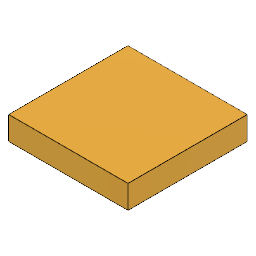
Post it Plotter v1 (Autodesk Fusion 360 archive; units mm, degrees)
design "Post It"
Autodesk Fusion 360 part; units mm, degrees
sketch "Skizze1" plane through (0, 0, 0) normal (0, 1, 0) x (1, 0, 0)
  line L0 (38.1, 38.1) -> (-38.1, 38.1)
  line L1 (-38.1, 38.1) -> (-38.1, -38.1)
  line L2 (-38.1, -38.1) -> (38.1, -38.1)
  line L3 (38.1, -38.1) -> (38.1, 38.1)
  line L4 (38.1, 38.1) -> (-38.1, -38.1) construction
  line L5 (-38.1, 38.1) -> (38.1, -38.1) construction
  dimension "d1" = 76.2
  dimension "d2" = 76.2
  constraint perpendicular L0 L1
  constraint parallel L0 L2
  constraint parallel L1 L3
  constraint horizontal L0
  constraint coincident L4 origin
  constraint coincident L5 origin
  measures "d1" distance of L1.end L2.end
  measures "d2" distance of L0.end L1.end
extrude "Extrusion1" add sketch "Skizze1" along normal blind 15 makes body 1
copy_body "Körper->Berechn1" bodies 1 removing the originals makes body 2 in component "Post It"
component "Post It" placed x (1, 0, 0) y (0, 1, 0) z (0, 0, 1) at (0, 0, 0)
named bodies: "Post It"

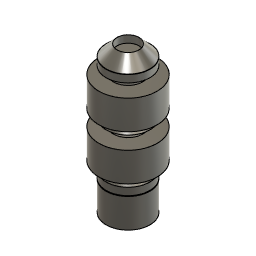
design "pivot"
Autodesk Fusion 360 part; units mm, degrees
sketch "Skizze1" plane through (0, 0, 0) normal (0, 1, 0) x (1, 0, 0)
  circle A0 centre (0, 0) radius 1.5
  circle A1 centre (0, 0) radius 4
  circle A2 centre (0, 0) radius 3
  dimension "d1" = 3
  dimension "d2" = 8
  dimension "d7" = 6
  constraint coincident A0.centre A1.centre
  constraint concentric A0 A1
  constraint concentric A1 A2
  measures "d1" diameter of A0
  measures "d2" diameter of A1
  measures "d7" diameter of A2
extrude "Extrusion1" add sketch "Skizze1" along normal blind 4 contours A1 | A2 makes body 1
extrude "Extrusion2" add sketch "Skizze1" against normal blind 4 separate body contours A1 | A2 makes body 2
move_body "Verschieben1" bodies 1 to x (1, 0, 0) y (0, 1, 0) z (0, 0, 1) at (0, 1, 0)
move_body "Verschieben2" bodies 2 to x (1, 0, 0) y (0, 1, 0) z (0, 0, 1) at (0, -1, 0)
extrude "Extrusion3" add sketch "Skizze1" along normal mid plane 2 separate body contours A2 makes body 3
copy_body "Körper kopieren/einfügen1" bodies 3 makes body 4
move_body "Verschieben3" bodies 4 to x (1, 0, 0) y (0, 1, 0) z (0, 0, 1) at (0, 6, 0)
copy_body "Körper kopieren/einfügen2" bodies 3 makes body 5
move_body "Verschieben4" bodies 5 to x (1, 0, 0) y (0, 1, 0) z (0, 0, 1) at (0, -6, 0)
chamfer "Fase1" distance 1 distance2 1 4 edges at (-2.797, 5, -1.0848) (-2.797, -5, 1.0848) (-2.797, -1, -1.0848) (-2.797, 1, 1.0848) measured on face at (2.4832, 5, 0.2236) measured on face at (2.4832, -5, 0.2236) measured on face at (2.4832, -1, 0.2236) measured on face at (2.4832, 1, 0.2236) on bodies 3 4 5
extrude "Extrusion4" add sketch "Skizze1" against normal blind 18.5 separate body contours A0 makes body 6
extrude "Extrusion5" add sketch "Skizze1" along normal blind 1.5 draft -45 contours A0 | A2 bodies 6
move_body "Verschieben6" bodies 6 to x (1, 0, 0) y (0, 1, 0) z (0, 0, 1) at (0, 7.2, 0)
extrude "Extrusion7" cut 1 faces at (0.4131, 8.7, 0.6492) along direction (0, -1, 0) blind 1 on bodies 6 bodies 6
extrude "Extrusion6" add sketch "Skizze1" against normal blind 4 separate body contours A2 makes body 7
move_body "Verschieben5" bodies 7 to x (1, 0, 0) y (0, 1, 0) z (0, 0, 1) at (0, -7.2, 0)
copy_body "Körper->Berechn1" bodies 1 removing the originals makes body 8 in component "bearing 1"
copy_body "Körper->Berechn2" bodies 2 removing the originals makes body 9 in component "bearing 2"
copy_body "Körper->Berechn3" bodies 3 removing the originals makes body 10 in component "spacer"
copy_body "Körper->Berechn4" bodies 4 removing the originals makes body 11 in component "spacer (1)"
copy_body "Körper->Berechn5" bodies 5 removing the originals makes body 12 in component "spacer (1) (1)"
copy_body "Körper->Berechn6" bodies 6 removing the originals makes body 13 in component "bolt"
copy_body "Körper->Berechn7" bodies 7 removing the originals makes body 14 in component "nut"
component "bearing 1" placed x (1, 0, 0) y (0, 1, 0) z (0, 0, 1) at (0, 0.05, 0)
component "bearing 2" placed x (1, 0, 0) y (0, 1, 0) z (0, 0, 1) at (0, -0.15, 0)
component "spacer" placed x (1, 0, 0) y (0, 1, 0) z (0, 0, 1) at (0, -0.05, 0)
component "spacer (1)" placed x (1, 0, 0) y (0, 1, 0) z (0, 0, 1) at (0, 0.15, 0)
component "spacer (1) (1)" placed x (1, 0, 0) y (0, 1, 0) z (0, 0, 1) at (0, -0.25, 0)
component "bolt" placed x (1, 0, 0) y (0, 1, 0) z (0, 0, 1) at (0, 0, 0)
component "nut" placed x (1, 0, 0) y (0, 1, 0) z (0, 0, 1) at (0, -0.15, 0)
named bodies: "bearing 1", "bearing 2", "spacer", "spacer (1)", "spacer (1) (1)", "bolt", "nut"

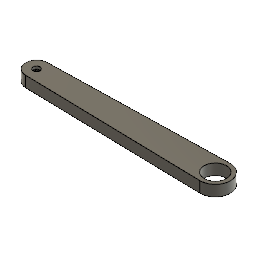
design "servo arm"
Autodesk Fusion 360 part; units mm, degrees
sketch "Skizze1" plane through (0, 0, 0) normal (0, 1, 0) x (1, 0, 0)
  line L0 (0, 0) -> (0, 2.5)
  line L1 (0, 0) -> (0.3428, 2.2743)
  line L2 (0, 0) -> (2.25, 0) construction
  line L3 (0, 2.5) -> (0.3428, 2.2743)
  line L4 (0, 2.5) -> (-0.3428, 2.2743)
  line L5 (0, 0) -> (-0.3428, 2.2743)
  line L6 (-0.7369, 2.3889) -> (-0.3428, 2.2743)
  line L7 (-0.7369, 2.3889) -> (-0.9979, 2.0722)
  line L8 (-1.4083, 2.0656) -> (-0.9979, 2.0722)
  line L9 (-1.4083, 2.0656) -> (-1.5644, 1.686)
  line L10 (-1.9546, 1.5587) -> (-1.5644, 1.686)
  line L11 (-1.9546, 1.5587) -> (-1.9919, 1.15)
  line L12 (-2.3272, 0.9134) -> (-1.9919, 1.15)
  line L13 (-2.3272, 0.9134) -> (-2.2423, 0.5118)
  line L14 (-2.493, 0.1868) -> (-2.2423, 0.5118)
  line L15 (-2.493, 0.1868) -> (-2.2936, -0.1719)
  line L16 (-2.4373, -0.5563) -> (-2.2936, -0.1719)
  line L17 (-2.4373, -0.5563) -> (-2.141, -0.8403)
  line L18 (-2.1651, -1.25) -> (-2.141, -0.8403)
  line L19 (-2.1651, -1.25) -> (-1.7982, -1.434)
  line L20 (-1.7004, -1.8326) -> (-1.7982, -1.434)
  line L21 (-1.7004, -1.8326) -> (-1.2956, -1.9003)
  line L22 (-1.0847, -2.2524) -> (-1.2956, -1.9003)
  line L23 (-1.0847, -2.2524) -> (-0.6779, -2.1978)
  line L24 (-0.3726, -2.4721) -> (-0.6779, -2.1978)
  line L25 (-0.3726, -2.4721) -> (0, -2.3)
  line L26 (0.3726, -2.4721) -> (0, -2.3)
  line L27 (0.3726, -2.4721) -> (0.6779, -2.1978)
  line L28 (1.0847, -2.2524) -> (0.6779, -2.1978)
  line L29 (1.0847, -2.2524) -> (1.2956, -1.9003)
  line L30 (1.7004, -1.8326) -> (1.2956, -1.9003)
  line L31 (1.7004, -1.8326) -> (1.7982, -1.434)
  line L32 (2.1651, -1.25) -> (1.7982, -1.434)
  line L33 (2.1651, -1.25) -> (2.141, -0.8403)
  line L34 (2.4373, -0.5563) -> (2.141, -0.8403)
  line L35 (2.4373, -0.5563) -> (2.2936, -0.1719)
  line L36 (2.493, 0.1868) -> (2.2936, -0.1719)
  line L37 (2.493, 0.1868) -> (2.2423, 0.5118)
  line L38 (2.3272, 0.9134) -> (2.2423, 0.5118)
  line L39 (2.3272, 0.9134) -> (1.9919, 1.15)
  line L40 (1.9546, 1.5587) -> (1.9919, 1.15)
  line L41 (1.9546, 1.5587) -> (1.5644, 1.686)
  line L42 (1.4083, 2.0656) -> (1.5644, 1.686)
  line L43 (1.4083, 2.0656) -> (0.9979, 2.0722)
  line L44 (0.7369, 2.3889) -> (0.9979, 2.0722)
  line L45 (0.7369, 2.3889) -> (0.3428, 2.2743)
  circle A0 centre (0, 0) radius 4
  circle A1 centre (65, 0) radius 4.05
  circle A2 centre (65, 0) radius 5.5
  line L46 (0.0212, 3.9999) -> (64.8729, 5.4985)
  line L47 (0.0212, -3.9999) -> (64.8729, -5.4985)
  circle A3 centre (0, 0) radius 1.25
  dimension "d1" = 2.5
  dimension "d2" = 81.429
  dimension "d3" = 2.3
  dimension "d5" = 360
  dimension "d6" = 8
  dimension "d7" = 8.1
  dimension "d8" = 65
  dimension "d9" = 11
  dimension "d14" = 2.5
  constraint coincident L0.start L1.start
  constraint vertical L0
  constraint horizontal L2
  constraint symmetric L3.start L0 L4.start
  constraint symmetric L0 L1.start L2.start
  constraint symmetric L0 L1.end L4.end
  constraint concentric A1 A2
  constraint coincident A0 L46.start
  constraint coincident A2 L46.end
  constraint tangent A2 L46
  constraint coincident A0 L47.start
  constraint coincident A2 L47.end
  constraint tangent A2 L47
  measures "d1" distance of L0.start L0.end
  measures "d2" angle of L1 L2
  measures "d3" distance of L0.start L1.end
  measures "d6" diameter of A0
  measures "d7" diameter of A1
  measures "d8" distance of L0.start A1.centre
  measures "d9" diameter of A2
  measures "d14" diameter of A3
extrude "Extrusion1" add sketch "Skizze1" against normal blind 4
extrude "Extrusion2" add sketch "Skizze1" against normal blind 1 contours L0 L4 L5 A3 | L0 L1 L3 A3 | L1 L5 L6 L7 L8 L9 L10 L11 L12 L13 L14 L15 L16 L17 L18 L19 L20 L21 L22 L23 L24 L25 L26 L27 L28 L29 L30 L31 L32 L33 L34 L35 L36 L37 L38 L39 L40 L41 L42 L43 L44 L45 A3
equation "d1 = ( ( 4.8 / 2 ) * 1 ) * 1 mm + 0.1 mm"
equation "d2 = 90 deg - ( 360 / 21 / 2 ) * 1 deg"
equation "d3 = ( ( 4.5 / 2 ) * 1 ) * 1 mm + 0.05 mm"
named bodies: "servo arm"

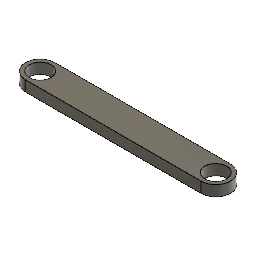
design "arm"
Autodesk Fusion 360 part; units mm, degrees
sketch "Skizze1" plane through (0, 0, 0) normal (0, 1, 0) x (1, 0, 0)
  circle A0 centre (-21.1614, -0.5404) radius 4.05
  circle A1 centre (43.8386, -0.5404) radius 4.05
  circle A2 centre (-21.1614, -0.5404) radius 5.5
  circle A3 centre (43.8386, -0.5404) radius 5.5
  line L0 (43.8386, 4.9596) -> (-21.1614, 4.9596)
  line L1 (-21.1614, -6.0404) -> (43.8386, -6.0404)
  dimension "d1" = 8.1
  dimension "d2" = 8.1
  dimension "d3" = 11
  dimension "d4" = 11
  dimension "d5" = 65
  constraint concentric A0 A2
  constraint concentric A1 A3
  constraint coincident A2 L0.end
  constraint tangent A2 L0
  constraint horizontal L0
  constraint coincident A3 L1.end
  constraint tangent A3 L1
  constraint parallel L0 L1
  constraint coincident A2 L1.start
  constraint tangent A2 L1
  constraint coincident A3 L0.start
  measures "d1" diameter of A0
  measures "d2" diameter of A1
  measures "d3" diameter of A2
  measures "d4" diameter of A3
  measures "d5" distance of A0.centre A1.centre
extrude "Extrusion1" add sketch "Skizze1" along normal blind 4
named bodies: "arm"

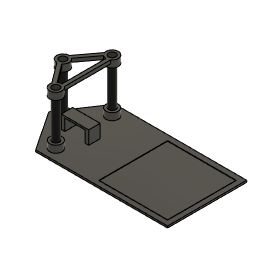
design "Base"
Autodesk Fusion 360 part; units mm, degrees
sketch "Skizze1" plane through (0, 0, 0) normal (0, 1, 0) x (1, 0, 0)
  line L0 (90, 45) -> (-60, 45)
  line L1 (-60, 45) -> (-60, -45)
  line L2 (-60, -45) -> (90, -45)
  line L3 (90, -45) -> (90, 45)
  line L4 (90, 45) -> (-60, -45) construction
  line L5 (-60, 45) -> (90, -45) construction
  line L6 (-60, 0) -> (-50, 0)
  circle A0 centre (-50, 32) radius 4.1
  circle A1 centre (-50, -32) radius 4.1
  circle A2 centre (-50, -32) radius 7
  circle A3 centre (-50, 32) radius 7
  line L7 (84, 39) -> (6, 39)
  line L8 (6, 39) -> (6, -39)
  line L9 (6, -39) -> (84, -39)
  line L10 (84, -39) -> (84, 39)
  line L11 (84, 39) -> (6, -39) construction
  line L12 (6, 39) -> (84, -39) construction
  line L13 (15, 0) -> (45, 0)
  line L14 (-60, 0) -> (-90, 0)
  line L15 (-60, 45) -> (-90, 0)
  line L16 (-60, -45) -> (-90, 0)
  circle A4 centre (-74, 0) radius 7
  circle A5 centre (-74, 0) radius 4.1
  line L17 (-74, 0) -> (-50, -32)
  line L18 (-50, 32) -> (-74, 0)
  line L19 (-50, 32) -> (-50, -32)
  line L20 (-43, 32) -> (-57, 32)
  line L21 (-43, -32) -> (-57, -32)
  line L22 (-46, 32) -> (-54, 32)
  line L23 (-54, 32) -> (-54, -32)
  line L24 (-54, -32) -> (-46, -32)
  line L25 (-46, -32) -> (-46, 32)
  line L26 (-46, 32) -> (-54, -32) construction
  line L27 (-54, 32) -> (-46, -32) construction
  line L28 (-74, 0) -> (-77.2, -2.4)
  line L29 (-74, 0) -> (-77.2, 2.4)
  line L30 (-74, 0) -> (-70.8, -2.4)
  line L31 (-74, 0) -> (-70.8, 2.4)
  line L32 (-70.8, 2.4) -> (-46.7262, -29.5318)
  line L33 (-77.2, -2.4) -> (-53.2861, -34.4518)
  line L34 (-70.8, -2.4) -> (-46.7262, 29.5318)
  line L35 (-77.2, 2.4) -> (-53.2861, 34.4518)
  point P0 (15, 0)
  point P1 (-50, 0)
  point P2 (-50, 0)
  point P3 (45, 0)
  point P4 (-50, 0)
  dimension "d1" = 150
  dimension "d2" = 90
  dimension "d3" = 10
  dimension "d6" = 8.2
  dimension "d7" = 8.2
  dimension "d8" = 14
  dimension "d9" = 14
  dimension "d15" = 78
  dimension "d16" = 78
  dimension "d17" = 30
  dimension "d26" = 30
  dimension "d27" = 14
  dimension "d28" = 8.2
  dimension "d29" = 8
  dimension "d30" = 4
  dimension "d31" = 4
  dimension "d32" = 4
  dimension "d33" = 4
  dimension "d62" = 90
  constraint perpendicular L0 L1
  constraint parallel L0 L2
  constraint parallel L1 L3
  constraint horizontal L0
  constraint coincident L4 P0
  constraint coincident L5 P0
  constraint midpoint L1 L6.start
  constraint perpendicular L1 L6
  constraint coincident P4 P2
  constraint concentric A1 A2
  constraint concentric A0 A3
  constraint perpendicular L7 L8
  constraint parallel L7 L9
  constraint parallel L8 L10
  constraint horizontal L7
  constraint coincident L11 P3
  constraint coincident L12 P3
  constraint coincident P0 L13.start
  constraint coincident P3 L13.end
  constraint horizontal L13
  constraint perpendicular L1 L14
  constraint coincident L14 A4.centre
  constraint concentric A4 A5
  constraint coincident A4.centre A5.centre
  constraint coincident A1.centre A2.centre
  constraint coincident A0.centre A3.centre
  constraint coincident A3 L20.start
  constraint coincident A3 L20.end
  constraint horizontal L20
  constraint coincident A2 L21.start
  constraint coincident A2 L21.end
  constraint parallel L20 L21
  constraint perpendicular L22 L23
  constraint parallel L22 L24
  constraint parallel L23 L25
  constraint horizontal L22
  constraint coincident L26 P4
  constraint coincident L27 P4
  constraint perpendicular L17 L28
  constraint perpendicular L18 L29
  constraint perpendicular L18 L30
  constraint perpendicular L17 L31
  constraint coincident A1 L32.end
  constraint tangent A1 L32
  constraint coincident A1 L33.end
  constraint tangent A1 L33
  constraint coincident A0 L34.end
  constraint tangent A0 L34
  constraint coincident A0 L35.end
  constraint tangent A0 L35
  measures "d1" distance of L1.end L2.end
  measures "d2" distance of L0.end L1.end
  measures "d3" distance of L6.start P4
  measures "d6" diameter of A0
  measures "d7" diameter of A1
  measures "d8" diameter of A2
  measures "d9" diameter of A3
  measures "d15" distance of L8.end L9.end
  measures "d16" distance of L7.end L8.end
  measures "d17" distance of P0 P3
  measures "d26" distance of L6.start L14.end
  measures "d27" diameter of A4
  measures "d28" diameter of A5
  measures "d29" distance of L23.end L24.end
  measures "d30" distance of A4.centre L28.end
  measures "d31" distance of A4.centre L29.end
  measures "d32" distance of A4.centre L30.end
  measures "d33" distance of A4.centre L31.end
  measures "d62" distance of origin L14.end
extrude "Extrusion1" add sketch "Skizze1" against normal blind 2 contours L0 L1 L2 L3 A2 A3 L25 L33 L35 | L1 L14 L15 A4 L35 | L1 A3 L18 L35 | L1 A4 L18 L35 | L1 L14 L16 A4 L33 | L1 A3 L18 L23 L34 | L1 A4 L18 L34 | L14 A4 A5 L35 | A4 A5 L18 L35 | A0 A3 L18 L20 L23 L35 | A3 L20 L35 | L14 A4 A5 L33 | L1 A4 L17 L33 | L1 A2 L17 L33 | L1 L6 L23 L34 | L1 L14 A4 L34 | A3 L18 L23 | A4 A5 L18 L32 L34 | L14 A5 L29 L35 | A5 L18 L29 L35 | A0 A3 L20 L35 | A0 L20 L35 | L14 A5 L28 L33 | A4 A5 L17 L33 | L1 A4 L17 L32 | L1 A2 L17 L23 L32 | A2 L21 L33 | A1 A2 L17 L21 L23 L33 | L1 L6 L23 L32 | L1 L14 A4 L32 | L14 A4 L34 | L6 A3 L19 L23 L34 | A3 L23 L34 | A0 A3 L18 L19 L23 L34 | A0 L18 L23 | A5 L18 L31 L32 | A0 A3 L20 L25 | A0 L20 L23 | A0 L20 L22 | L14 A5 L31 L32 | A5 L17 L30 L34 | A5 L17 L28 L33 | L14 A5 L30 L34 | A4 A5 L17 L32 L34 | A2 L17 L23 | A1 A2 L21 L33 | A1 L21 L33 | L6 A2 L19 L23 L32 | L14 A4 L32 | L14 A5 L34 | L14 A5 L32 | A3 L19 L34 | A0 L18 L19 | A0 L18 L20 L22 L23 | A2 A3 L19 L25 | A0 A3 L19 L25 L34 | A0 L20 L25 | A2 L23 L32 | A1 A2 L17 L19 L23 L32 | A1 L17 L23 | A1 A2 L21 L25 | A1 L21 L24 | A1 L21 L23 | A0 L19 L34 | A0 L19 L20 L22 L25 | A1 A2 L19 L25 L32 | A2 L19 L32 | A1 L17 L21 L23 L24 | A1 L17 L19 | A1 L21 L25 | A1 L19 L21 L24 L25 | A1 L19 L32 | L7 L8 L9 L10 makes body 1
extrude "Extrusion2" add sketch "Skizze1" along normal blind 8 contours L14 A4 A5 L35 | A4 A5 L18 L35 | A0 A3 L18 L20 L23 L35 | A3 L20 L35 | L14 A4 A5 L33 | A3 L18 L23 | A4 A5 L18 L32 L34 | A0 A3 L20 L35 | A0 L20 L35 | A4 A5 L17 L33 | A2 L21 L33 | A1 A2 L17 L21 L23 L33 | L14 A4 L34 | A0 A3 L18 L19 L23 L34 | A0 L18 L23 | A0 A3 L20 L25 | A4 A5 L17 L32 L34 | A2 L17 L23 | A1 A2 L21 L33 | A1 L21 L33 | L14 A4 L32 | L14 A5 L34 | L14 A5 L32 | A3 L19 L34 | A0 A3 L19 L25 L34 | A1 A2 L17 L19 L23 L32 | A1 L17 L23 | A1 A2 L21 L25 | A0 L19 L34 | A1 A2 L19 L25 L32 | A2 L19 L32 | A1 L19 L32 bodies 1
extrude "Extrusion3" cut sketch "Skizze1" against normal blind 0.5 contours L7 L8 L9 L10 bodies 1
sketch "Skizze5" plane through (0, 0, 0) normal (0, 1, 0) x (1, 0, 0)
  line L0 (-50, 32) -> (-74, 0)
  line L1 (-74, 0) -> (-50, -32)
  line L2 (-50, -32) -> (-50, 32)
  circle A0 centre (-50, 32) radius 4.1
  circle A1 centre (-50, 32) radius 7
  circle A2 centre (-74, 0) radius 4.1
  circle A3 centre (-74, 0) radius 7
  circle A4 centre (-50, -32) radius 4.1
  circle A5 centre (-50, -32) radius 7
  line L3 (-46, 32) -> (-54, 32)
  line L4 (-54, 32) -> (-54, -32)
  line L5 (-54, -32) -> (-46, -32)
  line L6 (-46, -32) -> (-46, 32)
  line L7 (-46, 32) -> (-54, -32) construction
  line L8 (-54, 32) -> (-46, -32) construction
  line L9 (-74, 0) -> (-78.8754, -4.8754)
  line L10 (-74, 0) -> (-67.0704, 0) construction
  line L11 (-74, 0) -> (-78.9497, 4.9497)
  line L12 (-74, 0) -> (-67, 0) construction
  line L13 (-76.8991, -2.8991) -> (-53.2826, -34.4566)
  line L14 (-76.8991, 2.8991) -> (-53.2826, 34.4566)
  line L15 (-74, 0) -> (-70.7174, -2.4566)
  line L16 (-74, 0) -> (-70.72, 2.46)
  line L17 (-70.72, 2.46) -> (-46.72, -29.54)
  line L18 (-70.7174, -2.4566) -> (-46.72, 29.54)
  point P0 (-50, 32)
  point P1 (-74, 0)
  point P2 (-50, -32)
  point P3 (-50, 0)
  dimension "d48" = 8.2
  dimension "d49" = 14
  dimension "d50" = 8.2
  dimension "d51" = 14
  dimension "d52" = 8.2
  dimension "d53" = 14
  dimension "d54" = 64
  dimension "d55" = 8
  dimension "d56" = 45
  dimension "d57" = 135
  constraint coincident P0 L0.start
  constraint coincident P1 L0.end
  constraint coincident P2 L1.end
  constraint perpendicular L3 L4
  constraint parallel L3 L5
  constraint parallel L4 L6
  constraint horizontal L3
  constraint coincident L7 P3
  constraint coincident L8 P3
  constraint midpoint L2 P3
  constraint horizontal L10
  constraint horizontal L12
  constraint coincident A2 L13.start
  constraint coincident L9 L13.start
  constraint coincident A4 L13.end
  constraint tangent A4 L13
  constraint coincident A2 L14.start
  constraint coincident L11 L14.start
  constraint coincident A0 L14.end
  constraint tangent A0 L14
  constraint coincident A2 L15.end
  constraint perpendicular L14 L15
  constraint coincident A2 L16.end
  constraint perpendicular L1 L16
  constraint coincident A4 L17.end
  constraint tangent A4 L17
  constraint coincident A0 L18.end
  constraint tangent A0 L18
  measures "d48" diameter of A0
  measures "d49" diameter of A1
  measures "d50" diameter of A2
  measures "d51" diameter of A3
  measures "d52" diameter of A4
  measures "d53" diameter of A5
  measures "d54" distance of L3.end L4.end
  measures "d55" distance of L4.end L5.end
  measures "d56" angle of L9 L10
  measures "d57" angle of L11 L12
extrude "Extrusion7" add sketch "Skizze5" along normal blind 4 separate body contours L0 L2 A0 A1 L4 L18 | L0 A0 L4 | L2 A0 L18 | L0 A1 L4 | L0 A0 A1 L4 L14 | L2 A0 A1 L6 L18 | L2 A1 L18 | A0 A1 L6 L14 | L0 A1 A3 L14 | L2 A1 A5 L6 | L0 A2 A3 L17 L18 | L0 A2 A3 L14 | L2 A4 A5 L6 L17 | L2 A5 L17 | A4 A5 L6 L13 | A3 L17 L18 | A3 L11 L14 | L2 A4 L17 | L1 L2 A4 A5 L4 L17 | A2 L17 L18 | A2 A3 L11 L13 | L1 A2 A3 L17 L18 | L1 A5 L4 | L1 A3 A5 L13 | L1 A4 A5 L4 L13 | L1 A2 A3 L13 | L1 A4 L4 makes body 2
extrude "Extrusion8" add sketch "Skizze5" against normal blind 4 contours L0 L2 A0 A1 L4 L18 | L0 A0 L4 | L2 A0 L18 | L0 A1 L4 | L0 A0 A1 L4 L14 | L2 A0 A1 L6 L18 | L2 A1 L18 | A0 A1 L6 L14 | L0 A2 A3 L17 L18 | L0 A2 A3 L14 | L2 A4 A5 L6 L17 | L2 A5 L17 | A4 A5 L6 L13 | A3 L17 L18 | A3 L11 L14 | L2 A4 L17 | L1 L2 A4 A5 L4 L17 | A2 L17 L18 | A2 A3 L11 L13 | L1 A2 A3 L17 L18 | L1 A5 L4 | L1 A4 A5 L4 L13 | L1 A2 A3 L13 | L1 A4 L4 bodies 2
move_body "Verschieben2" bodies 2 to x (1, 0, 0) y (0, 1, 0) z (0, 0, 1) at (0, 56, 0)
extrude "Extrusion6" add sketch "Skizze1" along normal blind 60 separate body contours L14 A5 L29 L35 | A5 L18 L29 L35 | L14 A5 L28 L33 | A5 L18 L31 L32 | A0 L20 L23 | A0 L20 L22 | L14 A5 L31 L32 | A5 L17 L30 L34 | A5 L17 L28 L33 | L14 A5 L30 L34 | A0 L18 L19 | A0 L18 L20 L22 L23 | A0 L20 L25 | A1 L21 L24 | A1 L21 L23 | A0 L19 L20 L22 L25 | A1 L17 L21 L23 L24 | A1 L17 L19 | A1 L21 L25 | A1 L19 L21 L24 L25 makes body 3 at (-45.9204, 40, -32.4082) makes body 4 at (-45.9204, 40, 31.5918) makes body 5 at (-74.712, 20, -4.0377)
copy_body "Körper->Berechn1" bodies 5 removing the originals makes body 6 in component "beam3"
copy_body "Körper->Berechn2" bodies 4 removing the originals makes body 7 in component "beam2"
copy_body "Körper->Berechn3" bodies 3 removing the originals makes body 8 in component "beam1"
copy_body "Körper->Berechn4" bodies 2 removing the originals makes body 9 in component "Top"
copy_body "Körper->Berechn5" bodies 1 removing the originals makes body 10 in component "Base"
sketch "Skizze2" plane through (0, 0, 0) normal (0, 1, 0) x (-1, 0, 0)
  line L0 (-6, -39) -> (-84, -39)
  line L1 (-84, -39) -> (-84, 39)
  line L2 (-84, 39) -> (-6, 39)
  line L3 (-6, 39) -> (-6, -39)
  circle A0 centre (50, -32) radius 7
  line L4 (-90, 45) -> (-90, -45)
  line L5 (-90, -45) -> (60, -45)
  line L6 (60, -45) -> (90, 0)
  line L7 (90, 0) -> (60, 45)
  line L8 (60, 45) -> (-90, 45)
  circle A1 centre (50, 32) radius 7
  circle A2 centre (74, 0) radius 7
  line L9 (51.5, -11.6) -> (64.5, -11.6)
  line L10 (64.5, -11.6) -> (64.5, 11.6)
  line L11 (64.5, 11.6) -> (51.5, 11.6)
  line L12 (51.5, 11.6) -> (51.5, -11.6)
  line L13 (51.5, -11.6) -> (64.5, 11.6) construction
  line L14 (64.5, -11.6) -> (51.5, 11.6) construction
  line L15 (74, 0) -> (58, 0)
  line L16 (64.5, 11.6) -> (51.5, 11.6)
  line L17 (51.5, 11.6) -> (51.5, 15.6)
  line L18 (51.5, 15.6) -> (64.5, 15.6)
  line L19 (64.5, 15.6) -> (64.5, 11.6)
  line L20 (64.5, -11.6) -> (51.5, -11.6)
  line L21 (51.5, -11.6) -> (51.5, -15.6)
  line L22 (51.5, -15.6) -> (64.5, -15.6)
  line L23 (64.5, -15.6) -> (64.5, -11.6)
  point P0 (58, 0)
  dimension "d34" = 23.2
  dimension "d35" = 13
  dimension "d36" = 16
  dimension "d37" = 4
  dimension "d38" = 4
  constraint perpendicular L9 L10
  constraint parallel L9 L11
  constraint parallel L10 L12
  constraint horizontal L9
  constraint coincident L13 P0
  constraint coincident L14 P0
  constraint coincident A2.centre L15.start
  constraint coincident P0 L15.end
  constraint perpendicular L10 L15
  constraint horizontal L16
  constraint vertical L17
  constraint horizontal L18
  constraint vertical L19
  constraint horizontal L20
  constraint vertical L21
  constraint horizontal L22
  constraint vertical L23
  constraint coincident L12 L11.end
  constraint coincident L12 L9.start
  measures "d34" distance of L9.end L10.end
  measures "d35" distance of L10.end L11.end
  measures "d36" distance of A2.centre P0
  measures "d37" distance of L10.end L18.end
  measures "d38" distance of L9.end L22.end
extrude "Extrusion1'" add sketch "Skizze2" along normal blind 13.2 separate body contours L9 L20 L21 L22 L23 | L11 L16 L17 L18 L19 makes body 11 at (-55.8333, 4.4, -11.6) makes body 12 at (-60.1667, 4.4, 11.6) in component "Base"
sketch "Skizze4" plane through (0, 13.2, 0) normal (0, 1, 0) x (-1, 0, 0)
  line L0 (64.5, -15.6) -> (64.5, -11.6)
  line L1 (64.5, -11.6) -> (51.5, -11.6)
  line L2 (51.5, -11.6) -> (51.5, -15.6)
  line L3 (51.5, -15.6) -> (64.5, -15.6)
  line L4 (64.5, -15.6) -> (51.5, -15.6)
  line L5 (51.5, -15.6) -> (51.5, 15.6)
  line L6 (51.5, 15.6) -> (64.5, 15.6)
  line L7 (64.5, 15.6) -> (64.5, -15.6)
  point P0 (51.5, 15.6)
  constraint horizontal L4
  constraint vertical L5
  constraint horizontal L6
  constraint vertical L7
  constraint coincident L0.start L3.end
  constraint coincident P0 L5.end
extrude "Extrusion2'" add sketch "Skizze4" along normal blind 2 bodies 11 12 in component "Base"
move_body "Verschieben1" bodies 11 to x (0, 0, -1) y (0, 1, 0) z (1, 0, 0) at (-49.9, 0, -54.1) in component "Base"
combine "Kombinieren1" operation add target body 10 tool bodies 11 in component "Base"
component "beam3" placed x (1, 0, 0) y (0, 1, 0) z (0, 0, 1) at (0, 0, 0)
component "beam2" placed x (1, 0, 0) y (0, 1, 0) z (0, 0, 1) at (0, 0, 0)
component "beam1" placed x (1, 0, 0) y (0, 1, 0) z (0, 0, 1) at (0, 0, 0)
component "Top" placed x (1, 0, 0) y (0, 1, 0) z (0, 0, 1) at (0, 0, 0)
component "Base" placed x (1, 0, 0) y (0, 1, 0) z (0, 0, 1) at (0, 0, 0)
equation "d34 = 22.6 mm + 0.6 mm"
equation "d39 = 12.2 mm + 1 mm"
equation "d57 = 180 deg - 45 deg"
named bodies: "Base", "beam1", "beam2", "beam3", "Top", "Top (1)"

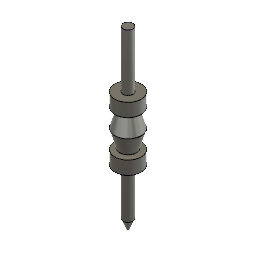
design "pen mount"
Autodesk Fusion 360 part; units mm, degrees
sketch "Skizze1" plane through (0, 0, 0) normal (0, 1, 0) x (1, 0, 0)
  circle A0 centre (0, 0) radius 1.5
  circle A1 centre (0, 0) radius 4
  dimension "d1" = 3
  dimension "d2" = 8
  constraint coincident A0.centre A1.centre
  constraint concentric A0 A1
  measures "d1" diameter of A0
  measures "d2" diameter of A1
extrude "Extrusion1" add sketch "Skizze1" along normal blind 4 makes body 1
extrude "Extrusion2" add sketch "Skizze1" along normal blind 50 and the other way blind 3 draft -22 separate body contours A0 makes body 2
move_body "Verschieben1" bodies 1 to x (1, 0, 0) y (0, 1, 0) z (0, 0, 1) at (0, 3, 0)
copy_body "Körper kopieren/einfügen1" bodies 1 makes body 3
move_body "Verschieben2" bodies 3 to x (1, 0, 0) y (0, 1, 0) z (0, 0, 1) at (0, 8.8, 0)
copy_body "Körper->Berechn1" bodies 1 removing the originals makes body 4 in component "bearing 1"
copy_body "Körper->Berechn2" bodies 2 removing the originals makes body 5 in component "pen"
copy_body "Körper->Berechn3" bodies 3 removing the originals makes body 6 in component "bearing 2"
sketch "Skizze2" plane through (0, 0, 0) normal (0, 1, 0) x (1, 0, 0)
  circle A0 centre (0, 0) radius 4
  circle A1 centre (0, 0) radius 1.5
  dimension "d49" = 8
  dimension "d50" = 3
  constraint coincident A0.centre A1.centre
  constraint concentric A0 A1
  measures "d49" diameter of A0
  measures "d50" diameter of A1
extrude "Extrusion3" add sketch "Skizze2" along normal mid plane 10.4 separate body makes body 7
chamfer "Fase1" distance 1.5 distance2 5.2 2 edges at (-3.7293, 5.2, 1.4465) (-3.7293, -5.2, -1.4465) measured on face at (3.1518, 5.2, 0.1987) measured on face at (3.1518, -5.2, 0.1987) on bodies 7
copy_body "Körper->Berechn4" bodies 7 removing the originals makes body 8 in component "spacer"
component "bearing 1" placed x (1, 0, 0) y (0, 1, 0) z (0, 0, 1) at (0, 26, 0)
component "pen" placed x (1, 0, 0) y (0, 1, 0) z (0, 0, 1) at (0, 0, 0)
component "bearing 2" placed x (1, 0, 0) y (0, 1, 0) z (0, 0, 1) at (0, 2.2, 0)
component "spacer" placed x (1, 0, 0) y (0, -1, 0) z (0, 0, -1) at (0, 23.5, 0)
named bodies: "bearing 1", "pen", "bearing 2", "spacer"
